Autodesk Inventor part; units mm, degrees
(part 2 of 2)
sketch "Sketch3" plane through (0, 0, 0) normal (0, 0, -1) x (-1, 0, 0)
  line L0 (0, 0) -> (-75.1754, 27.3616) construction
  line L1 (0, 0) -> (-66.0394, 45.153) construction
  line L2 (-75.1754, 27.3616) -> (-66.0394, 45.153) construction
  line L3 (0, 0) -> (-70, 0) construction
  arc A0 (-69.2544, 10.1895) -> (69.6176, 7.3067) centre (0, 0) ccw construction
  circle A1 centre (-75.1754, 27.3616) radius 4
  circle A2 centre (-66.0394, 45.153) radius 4
  circle A3 centre (1.6604, 79.9828) radius 17.5 construction
  circle A4 centre (0, 0) radius 17.5 construction
  arc A5 (61.3326, 86.2456) -> (-57.7006, 88.7167) centre (1.6604, 79.9828) ccw construction
  line L4 (-57.7006, 88.7167) -> (-69.2544, 10.1895) construction
  arc A6 (-69.2544, 10.1895) -> (69.6176, 7.3067) centre (0, 0) ccw construction
  line L5 (69.6176, 7.3067) -> (61.3326, 86.2456) construction
  line L6 (-62.4764, 16.2573) -> (-87.1754, 16.2573)
  line L7 (-87.1754, 16.2573) -> (-87.1754, 56.2573)
  line L8 (-87.1754, 56.2573) -> (-62.4764, 56.2573)
  line L9 (-62.4764, 56.2573) -> (-62.4764, 16.2573)
  line L10 (-62.4764, 16.2573) -> (-87.1754, 56.2573) construction
  line L11 (-87.1754, 16.2573) -> (-62.4764, 56.2573) construction
  point P0 (-74.8259, 36.2573)
  point P1 (-74.8259, 36.2573)
  point P2 (-70.6074, 36.2573)
  dimension "d8" = 80
  dimension "d9" = 20
  dimension "d10" = 20
  dimension "d11" = 8
  dimension "d12" = 40
  dimension "d13" = 12
  constraints: 20 end point, 4 midpoint, 2 centre point, 2 coincident, 2 horizontal, 2 parallel, 1 equal length, 1 equal radius, 1 horizontal alignment, 1 perpendicular, 1 point on circle, 1 point on line
  measures "d8" distance of L0.start L0.end
  measures "d9" distance of L0.end L1.end
  measures "d10" angle of L0 L3
  measures "d11" diameter of A1
  measures "d12" distance of L6.end L7.end
  measures "d13" distance from line of L0.end L7
extrude "Extrusion3" add sketch "Sketch3" against normal up to surface (12 mm away) contours A2 L9 L6 L7 L8
extrude "Extrusion5" [suppressed]
sketch "Sketch6" plane through (0, 0, 0) normal (0, 0, -1) x (-1, 0, 0)
  arc A0 (-63.6393, 48.353) -> (-64.6627, 41.3974) centre (-66.0394, 45.153) ccw projected
  line L0 (-63.6393, 48.353) -> (-64.6627, 41.3974) projected
  line L1 (-64.6627, 41.3974) -> (-63.6393, 48.353) projected
  circle A1 centre (-66.0394, 45.153) radius 4
  point P0 (0, 0)
  constraints: 1 coincident, 3 other
extrude "Extrusion6" cut sketch "Sketch6" against normal through all contours A1 L0
sketch "Sketch7" plane through (0, 0, 0) normal (0, 0, -1) x (-1, 0, 0)
  circle A0 centre (1.6604, 79.9828) radius 17.5 construction
  circle A1 centre (0, 0) radius 17.5 construction
  circle A2 centre (-66.0394, 45.153) radius 4 construction
  circle A3 centre (-75.1754, 27.3616) radius 4 construction
  line L0 (-68.3616, 16.2573) -> (-69.2544, 10.1895) construction
  arc A4 (-69.2544, 10.1895) -> (69.6176, 7.3067) centre (0, 0) ccw construction
  line L1 (69.6176, 7.3067) -> (61.3326, 86.2456) construction
  arc A5 (61.3326, 86.2456) -> (-57.7006, 88.7167) centre (1.6604, 79.9828) ccw construction
  line L2 (-57.7006, 88.7167) -> (-62.4764, 56.2573) construction
  line L3 (-87.1754, 56.2573) -> (-62.4764, 56.2573) construction
  line L4 (-87.1754, 16.2573) -> (-87.1754, 56.2573) construction
  line L5 (-68.3616, 16.2573) -> (-87.1754, 16.2573) construction
  arc A6 (-69.2544, 10.1895) -> (69.6176, 7.3067) centre (0, 0) ccw projected
  circle A7 centre (-69.2544, 10.1895) radius 2.159
  circle A8 centre (-1.4528, -69.9849) radius 2.159
  circle A9 centre (69.6176, 7.3067) radius 2.159
  arc A10 (61.3326, 86.2456) -> (-57.7006, 88.7167) centre (1.6604, 79.9828) ccw projected
  circle A11 centre (-57.7006, 88.7167) radius 2.159
  circle A12 centre (2.9056, 139.9698) radius 2.159
  line L6 (61.3326, 86.2456) -> (69.6176, 7.3067) projected
  circle A13 centre (61.3326, 86.2456) radius 2.159
  circle A14 centre (-69.2544, 10.1895) radius 4.5
  circle A15 centre (-1.4528, -69.9849) radius 4.5
  circle A16 centre (69.6176, 7.3067) radius 4.5
  circle A17 centre (61.3326, 86.2456) radius 4.5
  circle A18 centre (2.9056, 139.9698) radius 4.5
  line L7 (-62.4764, 56.2573) -> (-57.7006, 88.7167) projected
  circle A19 centre (-57.7006, 88.7167) radius 4.5
  dimension "d26" = 4.318
  dimension "d27" = 9
  constraints: 12 centre point, 10 equal radius, 8 coincident, 4 point on circle
  measures "d26" diameter of A7
  measures "d27" diameter of A14
extrude "Extrusion7" add sketch "Sketch7" against normal up to surface (12 mm away) contours A15 A6 A8 | A6 A8 A15 | A16 L6 A9 A6 | A6 A9 L6 A16 | A13 L6 A17 A10 | A10 A17 L6 A13 | A18 A10 A12 | A10 A12 A18 | A19 L7 A11 A10 | A10 A11 L7 A19 | A14
extrude "Extrusion8" cut sketch "Sketch7" against normal through all contours A8 A6 | A6 A8 | A9 L6 A6 | A6 L6 A9 | A7 | L6 A13 A10 | A10 A13 L6 | A12 A10 | A10 A12 | A11 L7 A10 | A10 L7 A11
sketch "Sketch8" plane through (0, 0, 12) normal (0, 0, 1) x (1, 0, 0)
  circle A0 centre (-69.6176, 7.3067) radius 2.159 construction
  circle A1 centre (69.2544, 10.1895) radius 2.159 construction
  arc A2 (-7.398, 139.7078) -> (-60.6954, 90.7003) centre (-1.6604, 79.9828) ccw construction
  arc A3 (-60.6954, 90.7003) -> (-61.8023, 81.7702) centre (-61.3326, 86.2456) ccw construction
  line L0 (-61.8023, 81.7702) -> (-69.1479, 11.7821) construction
  arc A4 (-69.1479, 11.7821) -> (-69.9432, 2.8185) centre (-69.6176, 7.3067) ccw construction
  arc A5 (-69.9432, 2.8185) -> (-3.0469, -69.9337) centre (0, 0) ccw construction
  arc A6 (-3.0469, -69.9337) -> (5.9465, -69.747) centre (1.4528, -69.9849) ccw construction
  arc A7 (5.9465, -69.747) -> (69.766, 5.7187) centre (0, 0) ccw construction
  arc A8 (69.766, 5.7187) -> (68.5994, 14.6416) centre (69.2544, 10.1895) ccw construction
  line L1 (68.5994, 14.6416) -> (68.3616, 16.2573) construction
  line L2 (87.1754, 16.2573) -> (68.3616, 16.2573) construction
  line L3 (87.1754, 56.2573) -> (87.1754, 16.2573) construction
  line L4 (62.4764, 56.2573) -> (87.1754, 56.2573) construction
  line L5 (62.4764, 56.2573) -> (58.3556, 84.2646) construction
  arc A9 (58.3556, 84.2646) -> (56.879, 93.141) centre (57.7006, 88.7167) ccw construction
  arc A10 (56.879, 93.141) -> (1.5937, 139.8945) centre (-1.6604, 79.9828) ccw construction
  arc A11 (1.5937, 139.8945) -> (-7.398, 139.7078) centre (-2.9056, 139.9698) ccw construction
  circle A12 centre (57.7006, 88.7167) radius 2.159 construction
  circle A13 centre (-2.9056, 139.9698) radius 2.159 construction
  circle A14 centre (-61.3326, 86.2456) radius 2.159 construction
  circle A15 centre (1.4528, -69.9849) radius 2.159 construction
  circle A16 centre (75.1754, 27.3616) radius 4 construction
  circle A17 centre (66.0394, 45.153) radius 4 construction
  line L6 (87.1754, 36.2573) -> (69.1754, 36.2573) construction
  line L7 (55.1754, 19.7573) -> (83.1754, 19.7573) construction
  line L8 (83.1754, 19.7573) -> (83.1754, 52.7573) construction
  line L9 (83.1754, 52.7573) -> (55.1754, 52.7573) construction
  line L10 (55.1754, 52.7573) -> (55.1754, 19.7573) construction
  line L11 (55.1754, 19.7573) -> (83.1754, 52.7573) construction
  line L12 (83.1754, 19.7573) -> (55.1754, 52.7573) construction
  circle A18 centre (83.1754, 52.7573) radius 1.397
  circle A19 centre (83.1754, 19.7573) radius 1.397
  circle A20 centre (55.1754, 19.7573) radius 1.397
  circle A21 centre (55.1754, 52.7573) radius 1.397
  dimension "d32" = 2.794
  dimension "d33" = 4
  dimension "d34" = 33
  dimension "d35" = 28
  constraints: 14 end point, 4 centre point, 4 coincident, 3 equal radius, 3 midpoint, 2 horizontal, 2 parallel, 1 perpendicular
  measures "d32" diameter of A18
  measures "d33" distance between parallel lines of L3 L8
  measures "d34" distance of L7.end L8.end
  measures "d35" distance of L8.end L9.end
extrude "Extrusion9" cut sketch "Sketch8" against normal through all
sketch "Sketch9" plane through (0, 0, 0) normal (0, 0, -1) x (-1, 0, 0)
  circle A0 centre (-55.1754, 19.7573) radius 1.397 projected
  circle A1 centre (-83.1754, 52.7573) radius 1.397 projected
  circle A2 centre (-83.1754, 19.7573) radius 1.397 projected
  circle A3 centre (-55.1754, 52.7573) radius 1.397 projected
  circle A4 centre (2.9056, 139.9698) radius 2.159 projected
  circle A5 centre (-1.4528, -69.9849) radius 2.159 projected
  circle A6 centre (61.3326, 86.2456) radius 2.159 projected
  circle A7 centre (-57.7006, 88.7167) radius 2.159 projected
  arc A8 (7.398, 139.7078) -> (-1.5937, 139.8945) centre (2.9056, 139.9698) ccw projected
  arc A9 (-1.5937, 139.8945) -> (-56.879, 93.141) centre (1.6604, 79.9828) ccw projected
  arc A10 (-56.879, 93.141) -> (-58.3556, 84.2646) centre (-57.7006, 88.7167) ccw projected
  line L0 (-58.3556, 84.2646) -> (-62.4764, 56.2573) projected
  line L1 (-87.1754, 56.2573) -> (-62.4764, 56.2573) projected
  line L2 (-87.1754, 16.2573) -> (-87.1754, 56.2573) projected
  line L3 (-68.3616, 16.2573) -> (-87.1754, 16.2573) projected
  line L4 (-68.3616, 16.2573) -> (-68.5994, 14.6416) projected
  arc A11 (-68.5994, 14.6416) -> (-69.766, 5.7187) centre (-69.2544, 10.1895) ccw projected
  arc A12 (-69.766, 5.7187) -> (-5.9465, -69.747) centre (0, 0) ccw projected
  arc A13 (-5.9465, -69.747) -> (3.0469, -69.9337) centre (-1.4528, -69.9849) ccw projected
  arc A14 (3.0469, -69.9337) -> (69.9432, 2.8185) centre (0, 0) ccw projected
  arc A15 (69.9432, 2.8185) -> (69.1479, 11.7821) centre (69.6176, 7.3067) ccw projected
  line L5 (69.1479, 11.7821) -> (61.8023, 81.7702) projected
  arc A16 (61.8023, 81.7702) -> (60.6954, 90.7003) centre (61.3326, 86.2456) ccw projected
  arc A17 (60.6954, 90.7003) -> (7.398, 139.7078) centre (1.6604, 79.9828) ccw projected
  circle A18 centre (-69.2544, 10.1895) radius 2.159 projected
  circle A19 centre (69.6176, 7.3067) radius 2.159 projected
  circle A20 centre (1.6604, 79.9828) radius 17.5 projected
  circle A21 centre (0, 0) radius 17.5 projected
  circle A22 centre (-66.0394, 45.153) radius 4 projected
  circle A23 centre (-75.1754, 27.3616) radius 4 projected
  line L6 (-87.1754, 16.2573) -> (-73.3182, 8.2569)
  arc A24 (-68.5994, 14.6416) -> (-69.766, 5.7187) centre (-69.2544, 10.1895) ccw projected
  dimension "d38" = 30
  constraints: 2 end point, 2 point on circle
  measures "d38" angle of L3 L6
ref_plane "Work Plane2" through (48.3454, 15.3651, 12) normal (0, 0, -1) x (0, 1, 0)
extrude "Extrusion10" add sketch "Sketch9" against normal up to surface (12 mm away) contours L3 L4 A11 L6
sketch "Sketch10" plane through (0, 0, 12) normal (0, 0, 1) x (1, 0, 0)
  line L0 (-130.7584, 64.7011) -> (20.7847, 170.8128)
  line L1 (20.7847, 170.8128) -> (134.3528, 8.6206)
  line L2 (134.3528, 8.6206) -> (-17.1903, -97.491)
  line L3 (-17.1903, -97.491) -> (-130.7584, 64.7011)
  arc A0 (-3.0469, -69.9337) -> (5.9465, -69.747) centre (1.4528, -69.9849) ccw projected
  arc A1 (-7.398, 139.7078) -> (-60.6954, 90.7003) centre (-1.6604, 79.9828) ccw projected
  arc A2 (-69.9432, 2.8185) -> (-3.0469, -69.9337) centre (0, 0) ccw projected
  line L4 (87.1754, 56.2573) -> (87.1754, 16.2573) projected
  arc A3 (5.9465, -69.747) -> (69.766, 5.7187) centre (0, 0) ccw projected
  dimension "d41" = 198
  dimension "d42" = 185
  dimension "d43" = 35
  constraints: 8 end point, 2 parallel, 2 tangent, 1 perpendicular
  measures "d41" distance of L2.end L0.start
  measures "d42" distance of L0.start L0.end
  measures "d43" angle of L1 L4
sketch "Sketch11" plane through (0, 0, 0) normal (0, 0, -1) x (-1, 0, 0)
  circle A0 centre (-55.1754, 19.7573) radius 1.397 projected
  circle A1 centre (-83.1754, 52.7573) radius 1.397 projected
  circle A2 centre (-83.1754, 19.7573) radius 1.397 projected
  circle A3 centre (-55.1754, 52.7573) radius 1.397 projected
  circle A4 centre (2.9056, 139.9698) radius 2.159 projected
  circle A5 centre (-1.4528, -69.9849) radius 2.159 projected
  circle A6 centre (61.3326, 86.2456) radius 2.159 projected
  circle A7 centre (-57.7006, 88.7167) radius 2.159 projected
  arc A8 (7.398, 139.7078) -> (-1.5937, 139.8945) centre (2.9056, 139.9698) ccw projected
  arc A9 (-1.5937, 139.8945) -> (-56.879, 93.141) centre (1.6604, 79.9828) ccw projected
  arc A10 (-56.879, 93.141) -> (-58.3556, 84.2646) centre (-57.7006, 88.7167) ccw projected
  line L0 (-58.3556, 84.2646) -> (-62.4764, 56.2573) projected
  line L1 (-87.1754, 56.2573) -> (-62.4764, 56.2573) projected
  line L2 (-87.1754, 16.2573) -> (-87.1754, 56.2573) projected
  line L3 (-87.1754, 16.2573) -> (-73.3182, 8.2569) projected
  arc A11 (-73.3182, 8.2569) -> (-69.766, 5.7187) centre (-69.2544, 10.1895) ccw projected
  arc A12 (-69.766, 5.7187) -> (-5.9465, -69.747) centre (0, 0) ccw projected
  arc A13 (-5.9465, -69.747) -> (3.0469, -69.9337) centre (-1.4528, -69.9849) ccw projected
  arc A14 (3.0469, -69.9337) -> (69.9432, 2.8185) centre (0, 0) ccw projected
  arc A15 (69.9432, 2.8185) -> (69.1479, 11.7821) centre (69.6176, 7.3067) ccw projected
  line L4 (69.1479, 11.7821) -> (61.8023, 81.7702) projected
  arc A16 (61.8023, 81.7702) -> (60.6954, 90.7003) centre (61.3326, 86.2456) ccw projected
  arc A17 (60.6954, 90.7003) -> (7.398, 139.7078) centre (1.6604, 79.9828) ccw projected
  circle A18 centre (-69.2544, 10.1895) radius 2.159 projected
  circle A19 centre (69.6176, 7.3067) radius 2.159 projected
  circle A20 centre (1.6604, 79.9828) radius 17.5 projected
  circle A21 centre (0, 0) radius 17.5 projected
  circle A22 centre (-66.0394, 45.153) radius 4 projected
  circle A23 centre (-75.1754, 27.3616) radius 4 projected
  arc A24 (-21.1246, -4) -> (-4, -21.1246) centre (0, 0) ccw
  arc A25 (-64.8768, -4) -> (-4, -64.8768) centre (0, 0) ccw
  line L5 (-4, -64.8768) -> (-4, -21.1246)
  line L6 (-21.1246, -4) -> (-64.8768, -4)
  arc A26 (4, -21.1246) -> (21.1246, -4) centre (0, 0) ccw
  circle A27 centre (0, 0) radius 6.75 projected
  arc A28 (4, -64.8768) -> (64.8768, -4) centre (0, 0) ccw
  line L7 (4, -64.8768) -> (4, -21.1246)
  line L8 (21.1246, -4) -> (64.8768, -4)
  arc A29 (-4, 21.1246) -> (-21.1246, 4) centre (0, 0) ccw
  line L9 (-21.1246, 4) -> (-51.1754, 4)
  line L10 (-51.1754, 4) -> (-51.1754, 35.9914)
  line L11 (-51.1754, 35.9914) -> (-4, 35.9914)
  line L12 (-4, 35.9914) -> (-4, 21.1246)
  line L13 (0, 0) -> (1.6604, 79.9828) construction
  arc A30 (21.1246, 4) -> (4, 21.1246) centre (0, 0) ccw
  line L14 (21.1246, 4) -> (64.9372, 4)
  line L15 (64.9372, 4) -> (61.5796, 35.9914)
  line L16 (61.5796, 35.9914) -> (4, 35.9914)
  line L17 (4, 35.9914) -> (4, 21.1246)
  line L18 (69.1479, 11.7821) -> (61.8023, 81.7702) projected
  arc A31 (-2.3396, 101.1074) -> (-19.4643, 83.9828) centre (1.6604, 79.9828) ccw
  arc A32 (-2.3396, 134.8371) -> (-53.194, 83.9828) centre (1.6604, 79.9828) ccw
  line L19 (-19.4643, 83.9828) -> (-53.194, 83.9828)
  line L20 (-2.3396, 134.8371) -> (-2.3396, 101.1074)
  arc A33 (22.785, 83.9828) -> (5.6604, 101.1074) centre (1.6604, 79.9828) ccw
  arc A34 (56.5147, 83.9828) -> (5.6604, 134.8371) centre (1.6604, 79.9828) ccw
  line L21 (5.6604, 101.1074) -> (5.6604, 134.8371)
  line L22 (22.785, 83.9828) -> (56.5147, 83.9828)
  arc A35 (-19.4643, 75.9828) -> (-2.3396, 58.8581) centre (1.6604, 79.9828) ccw
  arc A36 (5.6604, 58.8581) -> (22.785, 75.9828) centre (1.6604, 79.9828) ccw
  line L23 (5.6604, 58.8581) -> (5.6604, 43.9914)
  line L24 (5.6604, 43.9914) -> (60.7399, 43.9914)
  line L25 (60.7399, 43.9914) -> (57.3823, 75.9828)
  line L26 (57.3823, 75.9828) -> (22.785, 75.9828)
  line L27 (-2.3396, 58.8581) -> (-2.3396, 43.9914)
  line L28 (-2.3396, 43.9914) -> (-51.1754, 43.9914)
  line L29 (-51.1754, 43.9914) -> (-51.1754, 75.9828)
  line L30 (-51.1754, 75.9828) -> (-19.4643, 75.9828)
  point P0 (0.8302, 39.9914)
  dimension "d45" = 4
  dimension "d46" = 4
  dimension "d47" = 4
  dimension "d48" = 5
  dimension "d49" = 4
  dimension "d50" = 4
  dimension "d51" = 4
  dimension "d52" = 5
  dimension "d53" = 4
  dimension "d54" = 4
  dimension "d55" = 4
  dimension "d56" = 4
  dimension "d57" = 4
  dimension "d58" = 5
  dimension "d59" = 4
  dimension "d60" = 4
  dimension "d61" = 4
  dimension "d62" = 4
  dimension "d63" = 4
  dimension "d64" = 4
  dimension "d65" = 4
  dimension "d66" = 5
  dimension "d67" = 4
  dimension "d68" = 4
  dimension "d69" = 4
  dimension "d70" = 5
  dimension "d71" = 4
  dimension "d72" = 4
  dimension "d73" = 5
  dimension "d74" = 4
  dimension "d75" = 4
  dimension "d76" = 4
  dimension "d77" = 4
  dimension "d78" = 4
  dimension "d79" = 4
  constraints: 50 end point, 25 point on circle, 12 centre point, 12 coincident, 8 perpendicular, 7 horizontal, 5 vertical, 4 parallel, 1 midpoint
  measures "d45" distance from line of point (0, 0) L5
  measures "d46" distance from line of point (0, 0) L6
  measures "d47" radial gap between concentric circles of A21 A24
  measures "d48" radial gap between concentric circles of A12 A25
  measures "d49" distance from line of point (0, 0) L7
  measures "d50" distance from line of point (0, 0) L8
  measures "d51" radial gap between concentric circles of A21 A26
  measures "d52" radial gap between concentric circles of A14 A28
  measures "d53" distance from line of point (0.83, 39.991) L11
  measures "d54" radial gap between concentric circles of A21 A29
  measures "d55" distance from line of point (0, 0) L9
  measures "d56" distance from line of A0.centre L10
  measures "d57" distance from line of point (0, 0) L12
  measures "d58" distance between parallel lines of L4 L15
  measures "d59" distance from line of A21.centre L14
  measures "d60" radial gap between concentric circles of A21 A30
  measures "d61" distance from line of point (0, 0) L17
  measures "d62" distance from line of point (0.83, 39.991) L16
  measures "d63" distance from line of A32.centre L19
  measures "d64" radial gap between concentric circles of A20 A31
  measures "d65" distance from line of A9.centre L20
  measures "d66" radial gap between concentric circles of A9 A32
  measures "d67" distance from line of A9.centre L21
  measures "d68" distance from line of A9.centre L22
  measures "d69" radial gap between concentric circles of A20 A33
  measures "d70" radial gap between concentric circles of A17 A34
  measures "d71" distance from line of A9.centre L23
  measures "d72" distance from line of point (0.83, 39.991) L24
  measures "d73" distance between parallel lines of L4 L25
  measures "d74" distance from line of A9.centre L26
  measures "d75" radial gap between concentric circles of A20 A36
  measures "d76" distance from line of A31.centre L27
  measures "d77" distance from line of point (0.83, 39.991) L28
  measures "d78" distance from line of A31.centre L30
  measures "d79" distance from line of A3.centre L29
extrude "Extrusion11" cut sketch "Sketch11" against normal up to surface (10 mm away) contours A24 L5 A25 L6 | A26 L8 A28 L7 | A29 L9 L10 L11 L12 | A30 L17 L16 L15 L14 | A31 L19 A32 L20 | A33 L21 A34 L22 | A35 L27 L28 L29 L30 | A36 L26 L25 L24 L23
body "Solid1"
